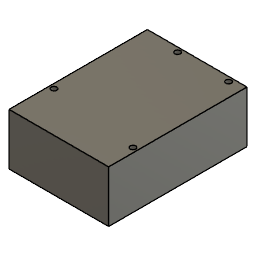
radartowrFinal (Autodesk Fusion 360 archive; units mm, degrees)
design "ARDUMODEL"
Autodesk Fusion 360 part; units mm, degrees
sketch "Sketch2" plane through (0, 0, 0) normal (0, 1, 0) x (1, 0, 0)
  line L0 (0, 0) -> (54, 0)
  line L1 (54, 0) -> (54, 75)
  line L2 (54, 75) -> (0, 75)
  line L3 (0, 75) -> (0, 0)
  circle A0 centre (46.5, 2.5) radius 1.5
  circle A1 centre (18.9, 2.5) radius 1.5
  circle A2 centre (51.5, 59.3) radius 1.5
  circle A3 centre (2.5, 53.1) radius 1.5
  dimension "d8" = 54
  dimension "d9" = 75
  dimension "d12" = 3
  dimension "d14" = 3
  dimension "d17" = 3
  dimension "d20" = 3
  constraint horizontal L0
  constraint vertical L1
  constraint horizontal L2
  constraint vertical L3
  constraint coincident L0.start L3.end
  measures "d8" distance of L0.start L0.end
  measures "d9" distance of L0.start L2.end
  measures "d12" diameter of A0
  measures "d14" diameter of A1
  measures "d17" diameter of A2
  measures "d20" diameter of A3
extrude "Extrude1" add sketch "Sketch2" along normal blind 28
move_body "Move1" bodies 1 to x (-1, 0, 0) y (0, 1, 0) z (0, 0, -1) at (54, 0, -75)
move_body "Move2" bodies 1 to x (-1, 0, 0) y (0, -1, 0) z (0, 0, 1) at (54, 28, 0)
